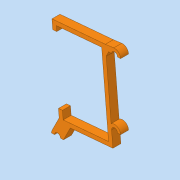
# Autodesk Inventor part: DriveBatteryHolder
Saved by Autodesk Inventor 2017 (Build 210142000, 142)
## iProperties
Created: 2018-01-30
Part Number: DriveBatteryHolder
Material: ABS Plastic
Document SubType Name: Modeling
Designer: Derek Wider
Density: 1.06 g/cm^3
Appearance: Orange
Author: Derek Wider
Autodesk Inventor part; units mm, degrees
ref_plane "YZ Plane" through (0, 0, 0) normal (1, 0, 0) x (0, 1, 0)
ref_plane "XZ Plane" through (0, 0, 0) normal (0, 1, 0) x (-1, 0, 0)
ref_plane "XY Plane" through (0, 0, 0) normal (0, 0, 1) x (1, 0, 0)
sketch "Sketch1" plane through (0, 0, 0) normal (0, 0, 1) x (1, 0, 0)
  arc A0 (1.905, 0) -> (-1.905, 0) centre (0, 0) ccw
  arc A1 (38.2001, 20.955) -> (34.3974, 20.789) centre (36.2951, 20.955) ccw
  arc A2 (38.2001, 62.865) -> (34.3901, 62.865) centre (36.2951, 62.865) ccw
  line L0 (32.4957, 13.3816) -> (3.6061, 10.8541)
  line L1 (32.4957, 13.3816) -> (61.4957, 13.3816) construction
  line L2 (32.4957, 13.3816) -> (28.1379, 63.1914)
  line L3 (28.1379, 63.1914) -> (-0.7517, 60.6639)
  line L4 (-3.5034, 62.9728) -> (30.4469, 65.9431)
  line L5 (31.0003, 59.6172) -> (35.2474, 11.0727)
  line L6 (35.2474, 11.0727) -> (8.1809, 8.7047)
  arc A3 (40.1051, 20.955) -> (34.1098, 24.076) centre (36.2951, 20.955) ccw
  line L7 (40.1051, 20.955) -> (38.2001, 20.955)
  arc A4 (38.2001, 20.955) -> (34.3974, 20.789) centre (36.2951, 20.955) ccw
  arc A5 (40.1051, 62.865) -> (35.8014, 66.6429) centre (36.2951, 62.865) ccw
  line L8 (30.4469, 65.9431) -> (35.8014, 66.6429)
  line L9 (34.3901, 62.865) -> (32.4851, 62.865)
  line L10 (32.4851, 62.865) -> (31.0003, 59.6172)
  line L11 (38.2001, 62.865) -> (40.1051, 62.865)
  arc A6 (-3.4049, 1.7097) -> (-3.81, 0) centre (0, 0) ccw
  line L12 (-1.905, 0) -> (-3.81, 0)
  line L13 (1.905, 0) -> (3.81, 0)
  line L14 (1.0757, 10.6327) -> (-3.4049, 1.7097)
  line L15 (3.81, 0) -> (8.1809, 8.7047)
  line L16 (-0.475, 57.5009) -> (-3.0053, 57.2796)
  line L17 (3.1633, 15.9148) -> (0.633, 15.6934)
  line L18 (-0.7517, 60.6639) -> (-0.475, 57.5009)
  line L19 (3.1633, 15.9148) -> (3.6061, 10.8541)
  line L20 (1.0757, 10.6327) -> (0.633, 15.6934)
  line L21 (-3.0053, 57.2796) -> (-3.5034, 62.9728)
  dimension "d0" = 3.81
  dimension "d1" = 3.81
  dimension "d2" = 3.81
  dimension "d3" = 41.91
  dimension "d4" = 41.91
  dimension "d5" = 120
  dimension "d6" = 175
  dimension "d7" = 29
  dimension "d8" = 50
  dimension "d9" = 2.54
  dimension "d10" = 7.62
  dimension "d11" = 3.81
  dimension "d12" = 6.35
  dimension "d13" = 7.62
  dimension "d14" = 5.08
  dimension "d15" = 3.175
  constraints: 44 end point, 14 point on circle, 7 centre point, 7 parallel, 6 perpendicular, 4 coincident, 4 horizontal, 4 point on line, 3 tangent, 1 concentric, 1 equal length, 1 horizontal alignment, 1 vertical alignment
  measures "d0" diameter of A0
  measures "d1" diameter of A1
  measures "d2" diameter of A2
  measures "d3" distance of A1.centre A2.centre
  measures "d4" distance of point (0, 0) A1.centre
  measures "d6" angle of L0 L1
  measures "d7" distance of L0.start L0.end
  measures "d8" distance of L0.start L2.end
  measures "d9" distance between parallel lines of L3 L4
  measures "d10" diameter of A5
  measures "d11" radius of A3
  measures "d12" distance of L5.start L4.end
  measures "d13" diameter of A6
  measures "d14" distance from line of L0.end L17
  measures "d15" distance between parallel lines of L16 L3
extrude "Extrusion1" add sketch "Sketch1" along normal blind 5.08
body "Solid1"
